Dryer Vibration Sensor (Autodesk Fusion 360 design; units mm, degrees)
Autodesk Fusion 360 part; units mm, degrees
sketch "Sketch1" plane through (0, 0, 0) normal (0, 0, 1) x (1, 0, 0)
  line L0 (0, 0) -> (29, 0)
  line L1 (29, 0) -> (29, 41)
  line L2 (29, 41) -> (0, 41)
  line L3 (0, 41) -> (0, 0)
  dimension "d1" = 29
  dimension "d2" = 41
  constraint horizontal L0
  constraint vertical L1
  constraint horizontal L2
  constraint vertical L3
  constraint coincident L0.start L3.end
  measures "d1" distance of L0.start L0.end
  measures "d2" distance of L0.start L2.end
extrude "Extrude1" add sketch "Sketch1" along normal blind 20 makes body 1
shell "Shell1" thickness 2 outward yes removed faces 1 at (9.6667, 27.3333, 20) on bodies 1
sketch "Sketch2" plane through (0, -2, 0) normal (0, -1, 0) x (1, 0, 0)
  line L0 (-2, -2) -> (31, -2)
  line L1 (31, -2) -> (31, 20)
  line L2 (31, 20) -> (-2, 20)
  line L3 (-2, 20) -> (-2, -2)
  line L4 (7, 18) -> (22, 18)
  line L5 (22, 18) -> (22, 10)
  line L6 (22, 10) -> (7, 10)
  line L7 (7, 10) -> (7, 18)
  dimension "d6" = 15
  dimension "d7" = 8
  dimension "d8" = 9
  dimension "d9" = 2
  constraint horizontal L4
  constraint vertical L5
  constraint horizontal L6
  constraint vertical L7
  measures "d6" distance of L4.start L4.end
  measures "d7" distance of L4.start L6.end
  measures "d8" distance of L3 L7
  measures "d9" distance of L2 L4
extrude "Extrude2" cut sketch "Sketch2" against normal blind 5 contours L4 L5 L6 L7 bodies 1
sketch "Sketch4" plane through (0, 0, 20) normal (0, 0, 1) x (-1, 0, 0)
  line L0 (0, -41) -> (-29, -41)
  line L1 (-29, -41) -> (-29, 0)
  line L2 (-29, 0) -> (0, 0)
  line L3 (0, 0) -> (0, -41)
  line L4 (2, -43) -> (2, 2)
  line L5 (2, 2) -> (-31, 2)
  line L6 (-31, 2) -> (-31, -43)
  line L7 (-31, -43) -> (2, -43)
  line L8 (2, -43) -> (-31, -43)
  line L9 (-31, -43) -> (-31, 2)
  line L10 (-31, 2) -> (2, 2)
  line L11 (2, 2) -> (2, -43)
  line L12 (0, -41) -> (-29, -41)
  line L13 (-29, -41) -> (-29, 0)
  line L14 (-29, 0) -> (0, 0)
  line L15 (0, 0) -> (0, -41)
  line L16 (-2, -39) -> (-27, -39)
  line L17 (-27, -39) -> (-27, -2)
  line L18 (-27, -2) -> (-2, -2)
  line L19 (-2, -2) -> (-2, -39)
  dimension "d12" = 2
  dimension "d13" = 2
  dimension "d14" = 2
  dimension "d15" = 2
  constraint horizontal L8
  constraint vertical L9
  constraint horizontal L10
  constraint vertical L11
  constraint coincident L5.end L6.start
  constraint coincident L4.start L7.end
  constraint horizontal L12
  constraint vertical L13
  constraint horizontal L14
  constraint vertical L15
  constraint coincident L1.end L2.start
  constraint coincident L0.start L3.end
  constraint horizontal L16
  constraint vertical L17
  constraint horizontal L18
  constraint vertical L19
  measures "d12" distance of L12 L16
  measures "d13" distance of L13 L17
  measures "d14" distance of L14 L18
  measures "d15" distance of L15 L19
extrude "Extrude3" add sketch "Sketch4" along normal blind 2 separate body contours L0 L1 L2 L3 L12 L13 L14 L15 | L4 L5 L6 L7 L8 L9 L10 L11 | L16 L17 L18 L19 makes body 2
extrude "Extrude4" add sketch "Sketch4" against normal blind 2 contours L0 L1 L2 L3 L12 L13 L14 L15 bodies 2
fillet "Fillet1" radius 0.75 4 edges at (7, -1, 10) (7, -1, 18) (22, -1, 10) (22, -1, 18) on bodies 1
hidden bodies 1
